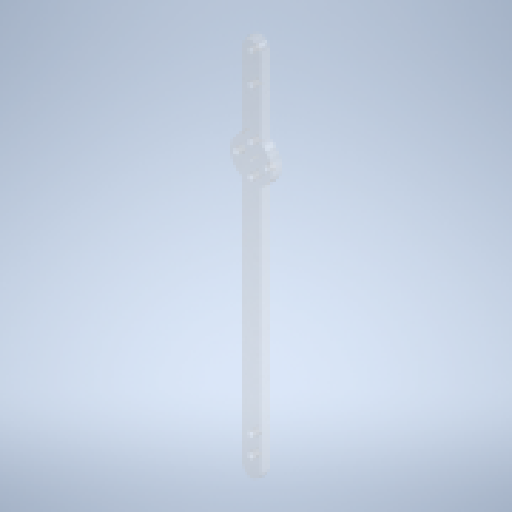
# Autodesk Inventor part: brazo
Saved by Autodesk Inventor 2023.1 (Build 271208000, 208)
## iProperties
Created: 2023-05-03
Part Number: brazo
Material: Acrylic
Document SubType Name: Modeling
Designer: felip
Density: 1.188 g/cm^3
Appearance: Transparent - Clear
Author: felip
Autodesk Inventor part; units mm, degrees
ref_plane "YZ Plane" through (0, 0, 0) normal (1, 0, 0) x (0, 1, 0)
ref_plane "XZ Plane" through (0, 0, 0) normal (0, 1, 0) x (-1, 0, 0)
ref_plane "XY Plane" through (0, 0, 0) normal (0, 0, 1) x (1, 0, 0)
sketch "Sketch1" plane through (0, 0, 0) normal (0, 0, 1) x (1, 0, 0)
  arc A0 (-5, 0) -> (5, 0) centre (0, 0) ccw
  arc A1 (5, 190) -> (-5, 190) centre (0, 190) ccw
  line L0 (-5, 190) -> (-5, 149.798)
  line L1 (-5, 130.202) -> (-5, 0)
  line L2 (5, 190) -> (5, 149.798)
  line L3 (5, 130.202) -> (5, 0)
  arc A2 (-5, 149.798) -> (-5, 130.202) centre (0, 140) ccw
  arc A3 (5, 130.202) -> (5, 149.798) centre (0, 140) ccw
  circle A4 centre (0, 190) radius 1.5
  circle A5 centre (0, 174) radius 1.5
  circle A6 centre (0, 5) radius 1.5
  circle A7 centre (0, 15) radius 1.5
  circle A8 centre (8, 140) radius 1.5
  circle A9 centre (0, 148) radius 1.5
  circle A10 centre (-8, 140) radius 1.5
  circle A11 centre (0, 132) radius 1.5
  dimension "d0" = 10
  dimension "d1" = 10
  dimension "d2" = 190
  dimension "d4" = 50
  dimension "d5" = 3
  dimension "d6" = 3
  dimension "d7" = 3
  dimension "d8" = 3
  dimension "d9" = 3
  dimension "d10" = 8
  dimension "d11" = 11
  dimension "d14" = 360
  dimension "d16" = 0
  dimension "d17" = 16
  dimension "d18" = 5
  dimension "d19" = 10
  dimension "d22" = 11
  constraints: 12 centre point, 8 end point, 8 point on circle, 6 tangent, 4 parallel, 2 coincident, 9 other
  measures "d0" diameter of A0
  measures "d1" diameter of A1
  measures "d2" distance of point (0, 0) A1.centre
  measures "d4" distance of A2.centre A1.centre
  measures "d5" diameter of A4
  measures "d6" diameter of A5
  measures "d7" diameter of A6
  measures "d8" diameter of A7
  measures "d9" diameter of A8
  measures "d10" distance of A8.centre A2.centre
  measures "d11" radius of A3
  measures "d16" distance of A1.centre A4.centre
  measures "d17" distance of A1.centre A5.centre
  measures "d18" distance of A0.centre A6.centre
  measures "d19" distance of A6.centre A7.centre
  measures "d22" radius of A2
extrude "Extrusion1" add sketch "Sketch1" along normal blind 5
move or copy body "Move Body1" bodies to move or copy 1 copy no translate (0, -140, 0)
sketch "Sketch3" plane through (0, -140, 5) normal (0, 0, 1) x (1, 0, 0)
  point P0 (0, 140)
equation "\"d5\" = d7"
equation "\"d6\" = d7"
equation "\"d8\" = d7"
equation "\"d22\" = d11"
body "Solid1"
